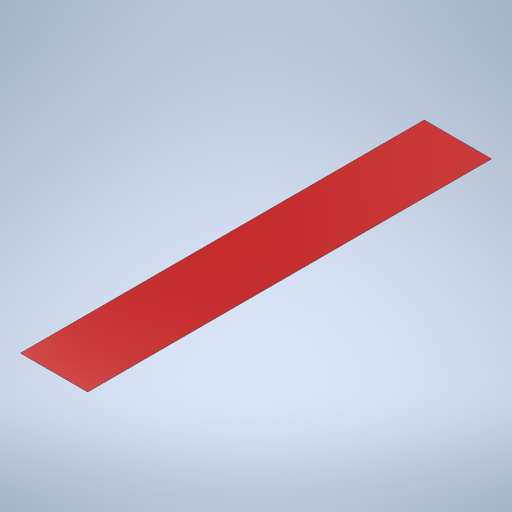
# Autodesk Inventor part: keepout - top A
Saved by Autodesk Inventor 2023 (Build 270158000, 158)
## iProperties
Created: 2023-03-02
Part Number: keepout - top A
Material: Generic
Document SubType Name: Modeling
Designer: Caleb
Density: 1 g/cm^3
Appearance: Default
Author: Caleb
Autodesk Inventor part; units mm, degrees
ref_plane "YZ Plane" through (0, 0, 0) normal (1, 0, 0) x (0, 1, 0)
ref_plane "XZ Plane" through (0, 0, 0) normal (0, 1, 0) x (-1, 0, 0)
ref_plane "XY Plane" through (0, 0, 0) normal (0, 0, 1) x (1, 0, 0)
sketch "Sketch1" plane through (0, 0, 0) normal (0, 1, 0) x (-1, 0, 0)
  line L0 (-2.5, -15) -> (2.5, -15)
  line L1 (2.5, -15) -> (2.5, 15)
  line L2 (2.5, 15) -> (-2.5, 15)
  line L3 (-2.5, 15) -> (-2.5, -15)
  line L4 (-2.5, -15) -> (2.5, 15) construction
  line L5 (2.5, -15) -> (-2.5, 15) construction
  point P0 (0, 0)
  dimension "d0" = 30
  dimension "d1" = 5
  constraints: 12 end point, 2 midpoint, 2 parallel, 1 horizontal, 1 perpendicular
  measures "d0" distance of L0.end L1.end
  measures "d1" distance of L1.end L2.end
extrude "Extrusion1" add sketch "Sketch1" along normal blind 0.01
body "Solid1"
